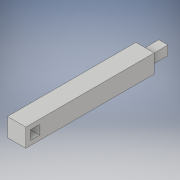
# Autodesk Inventor part: FrameAnalysisPart
Saved by Autodesk Inventor 2017 (Build 210142000, 142)
## iProperties
Created: 2018-03-23
Part Number: FrameAnalysisPart
Material: Generic
Document SubType Name: Modeling
Designer: User
Density: 1 g/cm^3
Appearance: Default
Author: User
Autodesk Inventor part; units mm, degrees
ref_plane "YZ Plane" through (0, 0, 0) normal (1, 0, 0) x (0, 1, 0)
ref_plane "XZ Plane" through (0, 0, 0) normal (0, 1, 0) x (-1, 0, 0)
ref_plane "XY Plane" through (0, 0, 0) normal (0, 0, 1) x (1, 0, 0)
sketch "Sketch1" plane through (0, 0, 0) normal (1, 0, 0) x (0, 1, 0)
  line L0 (0, 0) -> (25.4, 0)
  line L1 (25.4, 0) -> (25.4, -203.2)
  line L2 (25.4, -203.2) -> (0, -203.2)
  line L3 (0, -203.2) -> (0, 0)
  line L4 (19.05, -6.35) -> (6.35, -6.35)
  line L5 (6.35, -6.35) -> (6.35, -19.05)
  line L6 (6.35, -19.05) -> (19.05, -19.05)
  line L7 (19.05, -19.05) -> (19.05, -6.35)
  dimension "d0" = 25.4
  dimension "d1" = 203.2
  dimension "d2" = 12.7
  dimension "d3" = 12.7
  dimension "d4" = 6.35
  dimension "d5" = 6.35
  constraints: 16 end point, 4 parallel, 2 horizontal, 2 perpendicular
  measures "d0" distance of L1.end L2.end
  measures "d1" distance of L0.end L1.end
  measures "d2" distance of L6.end L5.end
  measures "d3" distance of L5.end L4.end
  measures "d4" distance between parallel lines of L1 L7
  measures "d5" distance between parallel lines of L0 L4
extrude "Extrusion1" add sketch "Sketch1" along normal blind 25.4
sketch "Sketch2" plane through (0, 0, -203.2) normal (0, 0, -1) x (-1, 0, 0)
  point P0 (0, 0)
sketch "Sketch3" plane through (0, 0, -203.2) normal (0, 0, -1) x (-1, 0, 0)
  line L0 (-19.05, 19.05) -> (-6.35, 19.05)
  line L1 (-6.35, 19.05) -> (-6.35, 6.35)
  line L2 (-6.35, 6.35) -> (-19.05, 6.35)
  line L3 (-19.05, 6.35) -> (-19.05, 19.05)
  line L4 (0, 25.4) -> (0, 0) projected
  line L5 (0, 25.4) -> (-25.4, 25.4) projected
  line L6 (-25.4, 0) -> (-25.4, 25.4) projected
  line L7 (0, 0) -> (-25.4, 0) projected
  dimension "d8" = 12.7
  dimension "d9" = 12.7
  dimension "d10" = 6.35
  dimension "d11" = 6.35
  constraints: 8 end point, 2 parallel, 1 horizontal, 1 perpendicular
  measures "d8" distance of L0.start L0.end
  measures "d9" distance of L0.end L1.end
  measures "d10" distance between parallel lines of L0 L5
  measures "d11" distance between parallel lines of L4 L1
extrude "Extrusion2" cut sketch "Sketch3" against normal blind 25.4
equation "\"d9\" = d8"
body "Solid1"
